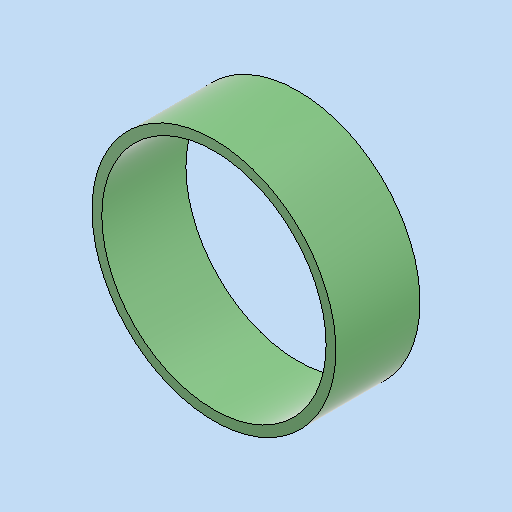
# Autodesk Inventor part: skirt-cylinder
Saved by Autodesk Inventor 2025 (Build 290162000, 162)
## iProperties
Created: 2024-10-31
Part Number: skirt-cylinder
Material: Stainless Steel
Document SubType Name: Modeling
Designer: kuzmin
Density: 8 g/cm^3
Appearance: Smooth - Dark Forest Green
Author: kuzmin
Autodesk Inventor part; units mm, degrees
ref_plane "YZ Plane" through (0, 0, 0) normal (1, 0, 0) x (0, 1, 0)
ref_plane "XZ Plane" through (0, 0, 0) normal (0, 1, 0) x (-1, 0, 0)
ref_plane "XY Plane" through (0, 0, 0) normal (0, 0, 1) x (1, 0, 0)
sketch "Sketch1" plane through (0, 0, 0) normal (1, 0, 0) x (0, 1, 0)
  line L0 (16, 6) -> (17.4, 6)
  line L1 (17.4, 6) -> (17.4, -6)
  line L2 (17.4, -6) -> (16, -6)
  line L3 (16, -6) -> (16, 6)
  line L4 (0, 0) -> (0, 17.75) construction
  point P0 (16, 0)
  dimension "d0" = 32
  dimension "d1" = 34.8
  dimension "d3" = 12
  constraints: 10 end point, 2 parallel, 1 horizontal, 1 horizontal alignment, 1 midpoint, 1 perpendicular, 1 vertical
  measures "d0" diameter of L3 L4
  measures "d1" diameter of L1 L4
  measures "d3" distance of L0.end L1.end
revolve "Revolution1" add sketch "Sketch1" angle 360 about axis through (0, 0, 0) along (0, 0, 1)
body "Solid1"
